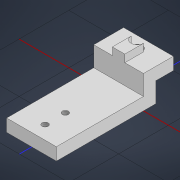
# Autodesk Inventor part: Nozzle_Brush_Holder_slim
Saved by Autodesk Inventor 2022 (Build 260153000, 153)
## iProperties
Created: 2022-02-27
Part Number: Nozzle_Brush_Holder_slim
Material: Generisch
Document SubType Name: Modeling
Designer: sleib
Density: 1 g/cm^3
Appearance: Vorgabe
Author: sleib
Autodesk Inventor part; units mm, degrees
ref_plane "YZ Plane" through (0, 0, 0) normal (1, 0, 0) x (0, 1, 0)
ref_plane "XZ Plane" through (0, 0, 0) normal (0, 1, 0) x (-1, 0, 0)
ref_plane "XY Plane" through (0, 0, 0) normal (0, 0, 1) x (1, 0, 0)
sketch "Skizze1" plane through (0, 0, 0) normal (1, 0, 0) x (0, 1, 0)
  line L0 (8, 0) -> (0, 0)
  line L1 (0, 0) -> (0, 35)
  line L2 (0, 35) -> (-5, 35)
  line L3 (-5, 35) -> (-5, -5)
  line L4 (-5, -5) -> (3, -5)
  line L5 (3, -5) -> (3, -12)
  line L6 (3, -12) -> (8, -12)
  line L7 (8, -12) -> (8, 0)
  dimension "d0" = 5
  dimension "d1" = 35
  dimension "d2" = 5
  dimension "d3" = 5
  dimension "d4" = 12
  dimension "d5" = 8
  constraints: 16 end point, 6 perpendicular, 1 horizontal, 1 vertical
  measures "d0" distance of L1.end L2.end
  measures "d1" distance between parallel lines of L0 L2
  measures "d2" distance between parallel lines of L4 L0
  measures "d3" distance between parallel lines of L7 L5
  measures "d4" distance of L6.end L0.start
  measures "d5" distance of L0.start L0.end
extrude "Extrusion1" add sketch "Skizze1" along normal mid plane 20
sketch "Skizze2" plane through (-10, 8, 0) normal (0, 1, 0) x (1, 0, 0)
  line L0 (20, 0) -> (0, 0) projected
  line L1 (12.5, 0) -> (7.5, 0)
  line L2 (7.5, 0) -> (7.5, 7.5)
  line L3 (7.5, 7.5) -> (12.5, 7.5)
  line L4 (12.5, 7.5) -> (12.5, 0)
  circle A0 centre (10, 7.5) radius 2.5
  point P0 (10, 0)
  point P1 (10, 0)
  dimension "d8" = 5
  dimension "d9" = 7.5
  dimension "d10" = 5
  constraints: 8 end point, 3 midpoint, 2 parallel, 1 centre point, 1 horizontal, 1 perpendicular, 1 point on line
  measures "d8" distance between parallel lines of L4 L2
  measures "d9" distance of L1.end L2.end
  measures "d10" diameter of A0
extrude "Extrusion2" add sketch "Skizze2" along normal blind 3 contours L0 L2 A0 L4
sketch "Skizze3" plane through (-10, 8, -12) normal (0, 1, 0) x (1, 0, 0)
  arc A0 (7.5, -4.5) -> (12.5, -4.5) centre (10, -4.5) ccw projected
  point P0 (10, -12)
  constraints: 1 coincident
hole "Bohrung1" at (0, 8, -7.5) direction (0, -1, 0) diameter 4.134 end through all thread size "M5x0.8" class "6H" standard "ISO Metric profile"
sketch "Skizze4" plane through (-10, 0, 35) normal (0, 1, 0) x (1, 0, 0)
  line L0 (10, 35) -> (10, 0) construction
  line L1 (0, 0) -> (20, 0) projected
  line L2 (20, 35) -> (0, 35) projected
  point P0 (10, 5.45)
  point P1 (10, 13.6)
  dimension "d20" = 21.4
  dimension "d21" = 29.55
  constraints: 2 end point, 2 point on line, 1 midpoint
  measures "d20" distance from line of point (10, 13.6) L2
  measures "d21" distance from line of point (10, 5.45) L2
hole "Bohrung2" at (0, 0, 29.55) at (0, 0, 21.4) direction (0, -1, 0) diameter 2.459 end through all thread size "M3x0.5" class "6H" standard "ISO Metric profile"
